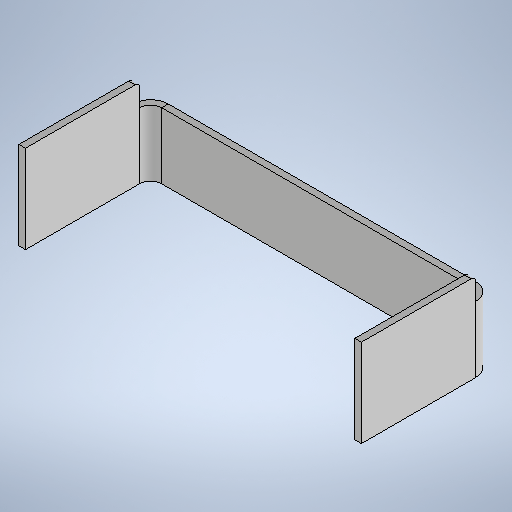
# Autodesk Inventor part: MSC 923 step
Saved by Autodesk Inventor 2025.1 (Build 291241020, 241B)
## iProperties
Created: 2024-07-01
Part Number: MSC 923 step
Material: Stainless Steel
Document SubType Name: Sheet Metal
Designer: user
Stock Number: МОО 902 опора рамы
Mass: 530.491 g
Surface Area: 354.574 cm^2
Volume: 66.3114 cm^3
Density: 8 g/cm^3
Flat Pattern Width: 4 cm
Flat Pattern Length: 26.3855 cm
Flat Pattern Area: 105.542 cm^2
Sheet Metal Rule: AISI304 3mm Die 32
Sheet Metal Width: 40.000 mm
Sheet Metal Length: 263.855 mm
Sheet Metal Area: 10554.195 mm^2
Appearance: Default
Author: pokla
Autodesk Inventor part; units mm, degrees
ref_plane "YZ Plane" through (0, 0, 0) normal (1, 0, 0) x (0, 1, 0)
ref_plane "XZ Plane" through (0, 0, 0) normal (0, 1, 0) x (-1, 0, 0)
ref_plane "XY Plane" through (0, 0, 0) normal (0, 0, 1) x (1, 0, 0)
sketch "Sketch1" plane through (0, 0, 0) normal (0, 1, 0) x (-1, 0, 0)
  line L0 (78, 15) -> (-78, 15)
  line L1 (-78, 15) -> (-78, -15)
  line L2 (-78, -15) -> (78, -15)
  line L3 (78, -15) -> (78, 15)
  line L4 (78, 15) -> (-78, -15) construction
  line L5 (-78, 15) -> (78, -15) construction
  point P0 (0, 0)
  dimension "d37" = 156
  dimension "d38" = 30
  measures "d37" distance of L2.end L1.end
  measures "d38" distance of L1.end L0.end
extrude "Plate1" add sketch "Sketch1" along normal blind 3
sketch "Sketch4" plane through (-75, 3, -15) normal (-1, 0, 0) x (0, -1, 0)
  line L0 (0, 30) -> (0, 0)
  line L1 (0, 0) -> (60, 0)
  line L2 (60, 0) -> (60, 30)
  line L3 (60, 30) -> (0, 30)
  constraints: 6 end point, 1 horizontal, 1 perpendicular, 1 vertical
edge flange "Flange1" height 60 angle 90 thickness 3 bend radius 5 thickness toward (-1, 0, 0) relief round relief width 3 relief depth 1.5 corner gap 5 corner form 0 edges at (-78, 0, 0) (78, 0, 0) wall of the first edge with corners at (-75, 3, 15) (-75, 3, -15) (-75, -57, -15) (-75, -57, 15)
bend "Bend1"
corner "Corner1"
sketch "Sketch5" plane through (-78, -57, 15) normal (0, 0, 1) x (1, 0, 0)
  line L0 (3, 52) -> (0, 52) projected
  line L1 (0, 52) -> (0, 0) projected
  line L2 (3, 0) -> (0, 0) projected
  line L3 (3, 52) -> (3, 0) projected
  point P0 (78, 57)
extrude "Extrusion2" add sketch "Sketch5" along normal blind 10
mirror "Mirror1" about plane through (0, 0, 0) normal (1, 0, 0) of "Extrusion2"
fillet "Fillet1" radius 2 2 edges at (76.5, -5, 25) (-76.5, -5, 25)
equation "\"d6\" = Thickness"
equation "\"d39\" = BendReliefWidth"
equation "\"d40\" = BendReliefDepth"
equation "\"d41\" = MinimumRemnant"
equation "\"d42\" = TransitionRadius"
equation "\"d45\" = BendRadius"
equation "\"d46\" = CornerReliefSize"
equation "\"d47\" = GapSize"
equation "\"d48\" = JacobiRadiusSize"
equation "\"BendReliefWidth\" = Thickness"
equation "\"BendReliefDepth\" = 0.5 * Thickness"
equation "\"CornerReliefSize\" = 4 * Thickness"
equation "\"MinimumRemnant\" = 2 * Thickness"
equation "\"TransitionRadius\" = BendRadius"
equation "\"JacobiRadiusSize\" = BendRadius"
equation "\"GapSize\" = Thickness"
equation "\"Thickness\" = 3"
equation "\"BendRadius\" = 5"
body "Solid1"
